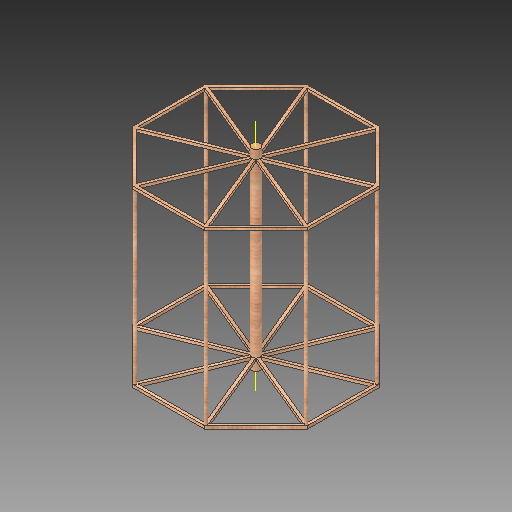
# Autodesk Inventor part: RuTAG Roller
Saved by Autodesk Inventor 2019 (Build 230136000, 136)
## iProperties
Created: 2019-05-13
Part Number: RuTAG Roller
Material: Wood (Birch)
Document SubType Name: Modeling
Designer: dell
Density: 0.55 g/cm^3
Appearance: Birch - Natural Polished
Author: dell
Autodesk Inventor part; units mm, degrees
ref_plane "YZ Plane" through (0, 0, 0) normal (1, 0, 0) x (0, 1, 0)
sketch "Sketch1" plane through (0, 0, 0) normal (0, 1, 0) x (-1, 0, 0)
  line L0 (-124.264069, -300) -> (-300, -124.264069)
  line L1 (-300, -124.264069) -> (-300, 124.264069)
  line L2 (-300, 124.264069) -> (-124.264069, 300)
  line L3 (-124.264069, 300) -> (124.264069, 300)
  line L4 (124.264069, 300) -> (300, 124.264069)
  line L5 (300, 124.264069) -> (300, -124.264069)
  line L6 (300, -124.264069) -> (124.264069, -300)
  line L7 (124.264069, -300) -> (-124.264069, -300)
  point P0 (0, 0)
  point P1 (0, 0)
  dimension "d0" = 600
  constraints: 16 end point, 1 coincident, 17 other
  measures "d0" distance between parallel lines of L1 L5
extrude "Extrusion1" add sketch "Sketch1" along normal blind 10
sketch "Sketch2" plane through (0, 10, 0) normal (0, 1, 0) x (1, 0, 0)
  point P0 (0, 0)
ref_plane "Work Plane1" through (0, -290, 0) normal (0, 1, 0) x (1, 0, 0)
mirror "Mirror1" about plane through (0, -290, 0) normal (0, 1, 0) of "Extrusion1"
sketch "Sketch6" plane through (0, 10, 0) normal (0, 1, 0) x (1, 0, 0)
  point P0 (0, 0)
shell "Shell3" thickness 10 removed faces 4 at (100, 10, 41.421356) at (100, -580, 41.421356) at (100, 0, 41.421356) at (100, -590, 41.421356)
sketch "Sketch7" plane through (0, 10, 0) normal (0, 1, 0) x (1, 0, 0)
  circle A0 centre (0, 0) radius 14.75
  dimension "d12" = 29.5
  constraints: 1 centre point, 1 coincident
  measures "d12" diameter of A0
extrude "Extrusion3" add sketch "Sketch7" along normal blind 30 and the other way blind 630
ref_plane "Work Plane3" through (120.121933, 0, 290) normal (-0.3826834, 0, 0.9238795) x (0, 1, 0)
sketch "Sketch8" plane through (120.121933, 0, 290) normal (-0.3826834, 0, 0.9238795) x (0, 1, 0)
  line L0 (0, 221.956391) -> (0, 0)
  line L1 (0, 443.912782) -> (0, 221.956391)
  line L2 (0, 221.956391) -> (10, 221.956391)
  line L3 (10, 221.956391) -> (10, 443.912782)
  line L4 (10, 0) -> (10, 221.956391)
  line L5 (10, 216.956391) -> (0, 216.956391)
  line L6 (0, 216.956391) -> (0, 226.956391)
  line L7 (0, 226.956391) -> (10, 226.956391)
  line L8 (10, 226.956391) -> (10, 216.956391)
  line L9 (10, 216.956391) -> (0, 226.956391) construction
  line L10 (0, 216.956391) -> (10, 226.956391) construction
  point P0 (5, 221.956391)
  dimension "d17" = 10
  dimension "d18" = 10
  constraints: 12 end point, 3 midpoint, 2 parallel, 1 horizontal, 1 perpendicular
  measures "d17" distance of L6.end L7.end
  measures "d18" distance of L5.end L6.end
extrude "Extrusion4" add sketch "Sketch8" along normal up to next
extrude "Extrusion5" add sketch "Sketch8" against normal up to next
pattern_circular "Circular Pattern1" count 8 over 360 about axis through (0, 40, 0) along (0, 1, 0) of "Extrusion4", "Extrusion5"
mirror "Mirror2" about plane through (0, -290, 0) normal (0, 1, 0) of "Extrusion4", "Extrusion5", "Circular Pattern1"
sketch "Sketch9" plane through (-124.264069, -580, -300) normal (0, 1, 0) x (1, 0, 0)
  line L0 (414.264069, -185.290028) -> (414.264069, -414.709972)
  line L1 (414.264069, -414.709972) -> (138.997875, -300.690981)
  arc A0 (135.171041, -309.929777) -> (138.997875, -300.690981) centre (124.264069, -300) ccw
  line L2 (410.437234, -423.948767) -> (135.171041, -309.929777)
  line L3 (410.437234, -423.948767) -> (248.212836, -586.173166)
  line L4 (248.212836, -586.173166) -> (134.193845, -310.906972)
  arc A1 (124.95505, -314.733806) -> (134.193845, -310.906972) centre (124.264069, -300) ccw
  line L5 (238.974041, -590) -> (124.95505, -314.733806)
  line L6 (238.974041, -590) -> (9.554097, -590)
  line L7 (9.554097, -590) -> (123.573087, -314.733806)
  arc A2 (114.334292, -310.906972) -> (123.573087, -314.733806) centre (124.264069, -300) ccw
  line L8 (0.315301, -586.173166) -> (114.334292, -310.906972)
  line L9 (0.315301, -586.173166) -> (-161.909097, -423.948767)
  line L10 (-161.909097, -423.948767) -> (113.357097, -309.929777)
  arc A3 (109.530263, -300.690981) -> (113.357097, -309.929777) centre (124.264069, -300) ccw
  line L11 (-165.735931, -414.709972) -> (109.530263, -300.690981)
  line L12 (-165.735931, -414.709972) -> (-165.735931, -185.290028)
  line L13 (-165.735931, -185.290028) -> (109.530263, -299.309019)
  arc A4 (113.357097, -290.070223) -> (109.530263, -299.309019) centre (124.264069, -300) ccw
  line L14 (-161.909097, -176.051233) -> (113.357097, -290.070223)
  line L15 (-161.909097, -176.051233) -> (0.315301, -13.826834)
  line L16 (0.315301, -13.826834) -> (114.334292, -289.093028)
  arc A5 (123.573087, -285.266194) -> (114.334292, -289.093028) centre (124.264069, -300) ccw
  line L17 (9.554097, -10) -> (123.573087, -285.266194)
  line L18 (9.554097, -10) -> (238.974041, -10)
  line L19 (238.974041, -10) -> (124.95505, -285.266194)
  arc A6 (134.193845, -289.093028) -> (124.95505, -285.266194) centre (124.264069, -300) ccw
  line L20 (248.212836, -13.826834) -> (134.193845, -289.093028)
  line L21 (248.212836, -13.826834) -> (410.437234, -176.051233)
  line L22 (410.437234, -176.051233) -> (135.171041, -290.070223)
  arc A7 (138.997875, -299.309019) -> (135.171041, -290.070223) centre (124.264069, -300) ccw
  line L23 (414.264069, -185.290028) -> (138.997875, -299.309019)
  line L24 (248.528137, 0) -> (424.264069, -175.735931)
  line L25 (0, 0) -> (248.528137, 0)
  line L26 (-175.735931, -175.735931) -> (0, 0)
  line L27 (-175.735931, -424.264069) -> (-175.735931, -175.735931)
  line L28 (0, -600) -> (-175.735931, -424.264069)
  line L29 (248.528137, -600) -> (0, -600)
  line L30 (424.264069, -424.264069) -> (248.528137, -600)
  line L31 (424.264069, -175.735931) -> (424.264069, -424.264069)
  arc A8 (109.530263, -300.690981) -> (113.357097, -309.929777) centre (124.264069, -300) ccw
  arc A9 (109.530263, -300.690981) -> (113.357097, -309.929777) centre (124.264069, -300) ccw
  arc A10 (113.357097, -290.070223) -> (109.530263, -299.309019) centre (124.264069, -300) ccw
  arc A11 (113.357097, -290.070223) -> (109.530263, -299.309019) centre (124.264069, -300) ccw
  arc A12 (123.573087, -285.266194) -> (114.334292, -289.093028) centre (124.264069, -300) ccw
  arc A13 (123.573087, -285.266194) -> (114.334292, -289.093028) centre (124.264069, -300) ccw
  arc A14 (134.193845, -289.093028) -> (124.95505, -285.266194) centre (124.264069, -300) ccw
  arc A15 (134.193845, -289.093028) -> (124.95505, -285.266194) centre (124.264069, -300) ccw
  arc A16 (138.997875, -299.309019) -> (135.171041, -290.070223) centre (124.264069, -300) ccw
  arc A17 (138.997875, -299.309019) -> (135.171041, -290.070223) centre (124.264069, -300) ccw
  arc A18 (135.171041, -309.929777) -> (138.997875, -300.690981) centre (124.264069, -300) ccw
  arc A19 (135.171041, -309.929777) -> (138.997875, -300.690981) centre (124.264069, -300) ccw
  arc A20 (124.95505, -314.733806) -> (134.193845, -310.906972) centre (124.264069, -300) ccw
  arc A21 (124.95505, -314.733806) -> (134.193845, -310.906972) centre (124.264069, -300) ccw
  arc A22 (114.334292, -310.906972) -> (123.573087, -314.733806) centre (124.264069, -300) ccw
  arc A23 (114.334292, -310.906972) -> (123.573087, -314.733806) centre (124.264069, -300) ccw
  arc A24 (109.530263, -300.690981) -> (113.357097, -309.929777) centre (124.264069, -300) ccw
  arc A25 (109.530263, -300.690981) -> (113.357097, -309.929777) centre (124.264069, -300) ccw
  arc A26 (113.357097, -290.070223) -> (109.530263, -299.309019) centre (124.264069, -300) ccw
  arc A27 (113.357097, -290.070223) -> (109.530263, -299.309019) centre (124.264069, -300) ccw
  arc A28 (123.573087, -285.266194) -> (114.334292, -289.093028) centre (124.264069, -300) ccw
  arc A29 (123.573087, -285.266194) -> (114.334292, -289.093028) centre (124.264069, -300) ccw
  arc A30 (134.193845, -289.093028) -> (124.95505, -285.266194) centre (124.264069, -300) ccw
  arc A31 (134.193845, -289.093028) -> (124.95505, -285.266194) centre (124.264069, -300) ccw
  arc A32 (138.997875, -299.309019) -> (135.171041, -290.070223) centre (124.264069, -300) ccw
  arc A33 (138.997875, -299.309019) -> (135.171041, -290.070223) centre (124.264069, -300) ccw
  arc A34 (135.171041, -309.929777) -> (138.997875, -300.690981) centre (124.264069, -300) ccw
  arc A35 (135.171041, -309.929777) -> (138.997875, -300.690981) centre (124.264069, -300) ccw
  arc A36 (124.95505, -314.733806) -> (134.193845, -310.906972) centre (124.264069, -300) ccw
  arc A37 (124.95505, -314.733806) -> (134.193845, -310.906972) centre (124.264069, -300) ccw
  arc A38 (114.334292, -310.906972) -> (123.573087, -314.733806) centre (124.264069, -300) ccw
  arc A39 (114.334292, -310.906972) -> (123.573087, -314.733806) centre (124.264069, -300) ccw
  circle A40 centre (124.264069, -300) radius 14.75
  circle A41 centre (124.264069, -300) radius 14.75
  arc A42 (134.193845, -289.093028) -> (124.95505, -285.266194) centre (124.264069, -300) ccw
  line L32 (124.264069, -300) -> (0, 0)
  line L33 (9.554097, -10) -> (123.573087, -285.266194)
  line L34 (9.554097, -10) -> (0.315301, -13.826834)
  circle A43 centre (2.564973, -6.192392) radius 6.192392
  circle A44 centre (2.564973, -6.192392) radius 5
  dimension "d26" = 10
  constraints: 4 end point, 3 tangent, 2 centre point, 1 coincident, 1 perpendicular, 1 other
  measures "d26" diameter of A44
extrude "Extrusion6" add sketch "Sketch9" along normal blind 580 contours A44 L32 | L32 A44
pattern_circular "Circular Pattern2" count 8 over 360 about axis through (0, 40, 0) along (0, 1, 0) of "Extrusion6"
body "Solid1"
